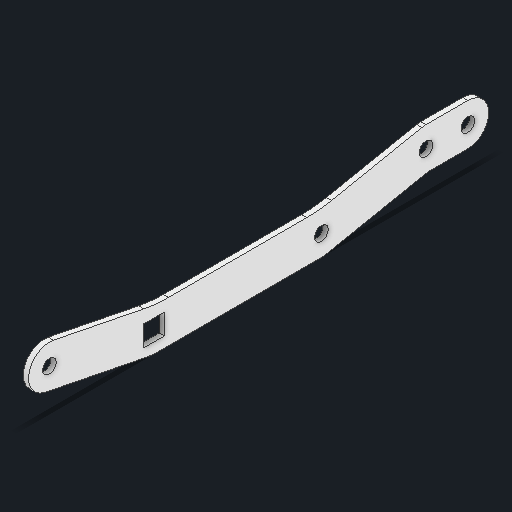
# Autodesk Inventor part: Conveyer Gearbox Gusset
Saved by Autodesk Inventor 2025.1 (Build 291241000, 241)
## iProperties
Created: 2024-11-21
Part Number: Conveyer Gearbox Gusset
Material: Acetal Resin, White
Document SubType Name: Modeling
Designer: avere
Density: 1.425 g/cm^3
Appearance: Smooth - White
Author: avere
Autodesk Inventor part; units mm, degrees
ref_plane "YZ Plane" through (0, 0, 0) normal (1, 0, 0) x (0, 1, 0)
ref_plane "XZ Plane" through (0, 0, 0) normal (0, 1, 0) x (-1, 0, 0)
ref_plane "XY Plane" through (0, 0, 0) normal (0, 0, 1) x (1, 0, 0)
sketch "Sketch1" plane through (0, 0, 0) normal (1, 0, 0) x (0, 1, 0)
  arc A0 (-2.5655, 28.8461) -> (-2.6888, 27.6008) centre (3.6612, 27.6008) ccw
  arc A1 (-2.6888, -23.1992) -> (-2.5655, -24.4445) centre (3.6612, -23.1992) ccw
  line L0 (-2.6888, 27.6008) -> (-2.6888, -23.1992)
  line L1 (10.0112, -18.7978) -> (10.0112, 23.1994)
  circle A2 centre (3.6612, -23.1992) radius 2.1082
  circle A3 centre (10.0112, 59.3508) radius 2.0955
  circle A4 centre (10.0112, -54.9492) radius 2.0955
  arc A5 (16.2378, 58.1055) -> (3.7845, 60.5961) centre (10.0112, 59.3508) ccw
  line L2 (3.7845, 60.5961) -> (-2.5655, 28.8461)
  line L3 (16.2378, 58.1055) -> (10.751, 30.6714)
  line L4 (3.6612, -55.578) -> (-2.5655, -24.4445)
  line L5 (16.2378, -53.7039) -> (10.751, -26.2698)
  arc A6 (10.751, 30.6714) -> (10.0112, 23.1994) centre (48.1112, 23.1994) ccw
  arc A7 (10.0112, -18.7978) -> (10.751, -26.2698) centre (48.1112, -18.7978) ccw
  line L6 (6.8108, 30.7504) -> (0.5116, 30.7504)
  line L7 (0.5116, 30.7504) -> (0.5116, 24.4512)
  line L8 (0.5116, 24.4512) -> (6.8108, 24.4512)
  line L9 (6.8108, 24.4512) -> (6.8108, 30.7504)
  line L10 (6.8108, 30.7504) -> (0.5116, 24.4512) construction
  line L11 (0.5116, 30.7504) -> (6.8108, 24.4512) construction
  arc A8 (3.6612, -67.6492) -> (16.3612, -67.6492) centre (10.0112, -67.6492) ccw
  line L12 (16.3612, -67.6492) -> (16.3612, -54.9492)
  line L13 (3.6612, -67.6492) -> (3.6612, -55.578)
  arc A9 (16.3612, -54.9492) -> (16.2378, -53.7039) centre (10.0112, -54.9492) ccw
  circle A10 centre (10.0112, -67.6492) radius 2.0955
  point P0 (0, 0)
  point P1 (10.0112, -22.5704)
  dimension "d0" = 12.7
  dimension "d1" = 12.7
  dimension "d3" = 4.2164
  dimension "d6" = 31.75
  dimension "d7" = 6.35
  dimension "d8" = 31.75
  dimension "d9" = 6.35
  dimension "d10" = 4.191
  dimension "d11" = 4.191
  dimension "d12" = 12.7
  dimension "d14" = 38.1
  dimension "d15" = 6.2992
  dimension "d16" = 6.2992
  dimension "d17" = 12.7
  dimension "d18" = 0
  dimension "d19" = 4.191
  constraints: 28 end point, 14 point on circle, 11 centre point, 9 tangent, 7 coincident, 5 parallel, 2 point on line, 1 equal radius, 1 horizontal, 1 perpendicular, 2 other
  measures "d0" diameter of A0
  measures "d1" diameter of A1
  measures "d3" diameter of A2
  measures "d6" vertical distance of point (10.011, -54.949) A1.centre
  measures "d7" horizontal distance of point (10.011, -54.949) A1.centre
  measures "d8" vertical distance of point (10.011, 59.351) A0.centre
  measures "d9" horizontal distance of A0.centre point (10.011, 59.351)
  measures "d10" diameter of A3
  measures "d11" diameter of A4
  measures "d12" diameter of A5
  measures "d14" radius of A6
  measures "d15" distance of L8.end L7.end
  measures "d16" distance of L7.end L6.end
  measures "d17" distance of point (10.011, -67.649) point (10.011, -54.949)
  measures "d18" horizontal distance of point (10.011, -67.649) A4.centre
  measures "d19" diameter of A10
extrude "Extrusion1" add sketch "Sketch1" along normal blind 1.5875
body "Solid1"
